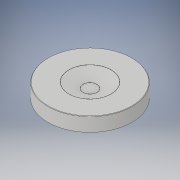
# Autodesk Inventor part: PARTE_SUPERIOR_BALSA_FLOTABILIDAD_UNIDMOTRIZVALPO
Saved by Autodesk Inventor 2019.4 (Build 234330000, 330)
## iProperties
Created: 2020-08-18
Part Number: PARTE_SUPERIOR_BALSA_FLOTABILIDAD_UNIDMOTRIZVALPO
Material: Generic
Document SubType Name: Modeling
Designer: crist
Density: 1 g/cm^3
Appearance: Default
Author: crist
Autodesk Inventor part; units mm, degrees
ref_plane "YZ Plane" through (0, 0, 0) normal (1, 0, 0) x (0, 1, 0)
ref_plane "XZ Plane" through (0, 0, 0) normal (0, 1, 0) x (-1, 0, 0)
ref_plane "XY Plane" through (0, 0, 0) normal (0, 0, 1) x (1, 0, 0)
sketch "Boceto1" plane through (0, 0, 0) normal (0, 0, 1) x (1, 0, 0)
  line L0 (0, 0) -> (0, 1000)
  line L1 (3000, 1000) -> (3000, 0)
  line L2 (3000, 0) -> (0, 0)
  line L3 (3000, 1000) -> (2000, 1000)
  line L4 (0, 600) -> (500, 600)
  line L5 (2000, 1000) -> (1500, 1000)
  line L6 (1500, 1000) -> (500, 600)
  dimension "d0" = 1000
  dimension "d1" = 3000
  dimension "d2" = 1000
  dimension "d4" = 500
  dimension "d5" = 500
  constraints: 14 end point, 1 perpendicular, 1 point on line, 1 vertical
  measures "d0" distance of L0.start L0.end
  measures "d1" distance of L0.end L1.start
  measures "d2" distance of L1.start L3.end
  measures "d4" distance of L4.start L4.end
  measures "d5" distance of L3.end L5.end
revolve "Revolución1" add sketch "Boceto1" angle 360 about axis through (0, 0, 0) along (0, 1, 0)
fillet "Empalme1" radius 30 1 edges at (-500, 600, 0)
fillet "Empalme2" radius 30 1 edges at (-1500, 1000, 0)
fillet "Empalme3" radius 30 1 edges at (-3000, 1000, 0)
